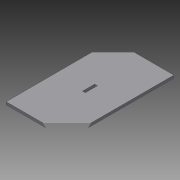
# Autodesk Inventor part: Base
Saved by Autodesk Inventor 2014 (Build 180170000, 170)
## iProperties
Created: 2015-02-09
Part Number: Base
Material: Generic
Document SubType Name: Modeling
Designer: ThatOtherGuy
Density: 1 g/cm^3
Appearance: Default
Author: ThatOtherGuy
Autodesk Inventor part; units mm, degrees
ref_plane "YZ Plane" through (0, 0, 0) normal (1, 0, 0) x (0, 1, 0)
ref_plane "XZ Plane" through (0, 0, 0) normal (0, 1, 0) x (-1, 0, 0)
ref_plane "XY Plane" through (0, 0, 0) normal (0, 0, 1) x (1, 0, 0)
sketch "Sketch1" plane through (0, 0, 0) normal (0, 0, 1) x (1, 0, 0)
  line L0 (0, 0) -> (200, 0)
  line L1 (200, 0) -> (200, 263.462)
  line L2 (200, 263.462) -> (0, 263.462)
  line L3 (0, 263.462) -> (0, 0)
  dimension "d0" = 200
  dimension "d1" = 263.462
  constraints: 8 end point, 2 parallel, 1 horizontal, 1 perpendicular
  measures "d0" distance of L0.start L0.end
  measures "d1" distance of L2.end L0.start
extrude "Extrusion1" add sketch "Sketch1" along normal blind 6.731
sketch "Sketch2" plane through (0, 0, 6.731) normal (0, 0, 1) x (1, 0, 0)
  line L0 (200, 263.462) -> (0, 263.462) projected
  line L1 (0, 263.462) -> (0, 0) projected
  line L2 (96.6345, 146.731) -> (103.3655, 146.731)
  line L3 (103.3655, 146.731) -> (103.3655, 116.731)
  line L4 (103.3655, 116.731) -> (96.6345, 116.731)
  line L5 (96.6345, 116.731) -> (96.6345, 146.731)
  point P0 (100, 146.731)
  point P1 (100, 263.462)
  point P2 (96.6345, 131.731)
  point P3 (0, 131.731)
  dimension "d4" = 30
  dimension "d5" = 6.731
  constraints: 8 end point, 4 midpoint, 2 parallel, 1 horizontal, 1 horizontal alignment, 1 perpendicular, 1 vertical alignment
  measures "d4" distance of L4.end L2.start
  measures "d5" distance of L2.start L2.end
extrude "Extrusion2" cut sketch "Sketch2" against normal up to next
equation "\"d2\" = THICKB"
equation "\"THICKA\" = 3.175"
equation "\"THICKB\" = 6.731"
equation "\"THICKC\" = 12.7"
equation "\"THICKPLY\" = 5"
equation "\"MAGDIA\" = 9.5"
equation "\"BALLDIA\" = 12"
body "Solid1"
